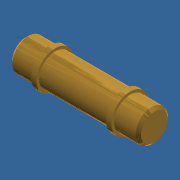
# Autodesk Inventor part: Welle 5x4+6x15+5x4
Saved by Autodesk Inventor 2016 (Build 200138000, 138)
## iProperties
Created: 2015-09-10
Part Number: Welle 5x4+6x15+5x4
Material: Messing, weicher Gelbton
Document SubType Name: Modeling
Designer: 4ndreas
Density: 8.47 g/cm^3
Appearance: Messing - satiniert
Mass: 6.67006 g
Surface Area: 5.92098 cm^2
Volume: 0.787493 cm^3
CustomPartVersion: 1
Author: 4ndreas
Autodesk Inventor part; units mm, degrees
ref_plane "Startebene" through (0, 0, 0) normal (1, 0, 0) x (0, 1, 0)
ref_plane "XZ Plane" through (0, 0, 0) normal (0, 1, 0) x (-1, 0, 0)
ref_plane "XY Plane" through (0, 0, 0) normal (0, 0, 1) x (1, 0, 0)
sketch "Hauptskizze" plane through (0, 0, 0) normal (0, 0, 1) x (1, 0, 0)
  line L0 (0, 0) -> (25, 0)
  line L1 (0, 0) -> (0, 2.5)
  line L2 (0, 2.5) -> (5, 2.5)
  line L3 (5, 2.5) -> (5, 4)
  line L4 (6, 4) -> (6, 3.5)
  line L5 (5, 4) -> (6, 4)
  line L6 (6, 3.5) -> (19, 3.5)
  line L7 (20, 4) -> (20, 2.5)
  line L8 (19, 4) -> (20, 4)
  line L9 (25, 2.5) -> (25, 0)
  line L10 (20, 2.5) -> (25, 2.5)
  line L11 (19, 3.5) -> (19, 4)
  dimension "d3" = 5
  dimension "d4" = 8
  dimension "d5" = 7
  dimension "d13" = 8
  dimension "d14" = 5
  constraints: 24 end point, 6 vertical, 1 horizontal
  measures "d3" diameter of L2 L0
  measures "d4" diameter of L5 L0
  measures "d5" diameter of L6 L0
  measures "d13" diameter of L8 L0
  measures "d14" diameter of L10 L0
revolve "Umdrehung1" add sketch "Hauptskizze" angle 360 about axis through (0, 0, 0) along (1, 0, 0)
chamfer "Fase5" distance 0.5 angle 45 1 edges at (19, -4, 0) measured on face at (19.3333, 3.987, -0.3219)
chamfer "Fase4" distance 0.5 angle 45 1 edges at (6, -4, 0) measured on face at (5.3333, 3.987, -0.3219)
chamfer "Fase3" distance 0.5 angle 45 1 edges at (25, -2.5, 0) measured on face at (21.6667, 2.4676, -0.401)
chamfer "Fase1" distance 0.5 angle 45 1 edges at (0, -2.5, 0) measured on face at (1.6667, 2.4676, -0.401)
